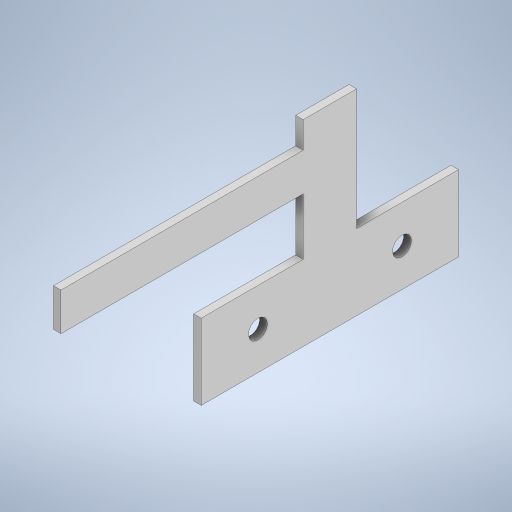
# Autodesk Inventor part: manual_locker_raw
Saved by Autodesk Inventor 2024 (Build 280153000, 153)
## iProperties
Created: 2025-12-30
Part Number: manual_locker_raw
Material: Generic
Document SubType Name: Modeling
Designer: schar
Density: 1 g/cm^3
Appearance: Default
Author: schar
Autodesk Inventor part; units mm, degrees
ref_plane "YZ Plane" through (0, 0, 0) normal (1, 0, 0) x (0, 1, 0)
ref_plane "XZ Plane" through (0, 0, 0) normal (0, 1, 0) x (-1, 0, 0)
ref_plane "XY Plane" through (0, 0, 0) normal (0, 0, 1) x (1, 0, 0)
sketch "Sketch1" plane through (0, 0, 0) normal (1, 0, 0) x (0, 1, 0)
  line L0 (10, 34.056) -> (-10, 34.056)
  line L1 (-10, 34.056) -> (-10, -34.056)
  line L2 (-10, -34.056) -> (10, -34.056)
  line L3 (10, -34.056) -> (10, 34.056)
  line L4 (10, 34.056) -> (-10, -34.056) construction
  line L5 (-10, 34.056) -> (10, -34.056) construction
  line L6 (10, 0) -> (10, -7.056)
  line L7 (10, -7.056) -> (42, -7.056)
  line L8 (42, -7.056) -> (42, 7.056)
  line L9 (42, 7.056) -> (10, 7.056)
  line L10 (10, 7.056) -> (10, -7.056)
  line L11 (0, 34.056) -> (0, 19.056)
  line L12 (0, -34.056) -> (0, -19.056)
  circle A0 centre (0, 19.056) radius 2.5
  circle A1 centre (0, -19.056) radius 2.5
  line L13 (10, 7.056) -> (10, 34.056)
  line L14 (10, 7.056) -> (10, 19.9232)
  line L15 (10, 19.9232) -> (25, 19.9232)
  line L16 (25, 19.9232) -> (25, 7.056)
  line L17 (25, 7.056) -> (10, 7.056)
  line L18 (25, 7.056) -> (25, 71.168)
  line L19 (25, 71.168) -> (35, 71.168)
  line L20 (35, 71.168) -> (35, 7.056)
  line L21 (35, 7.056) -> (25, 7.056)
  line L22 (35, 7.056) -> (35, 27.056)
  line L23 (35, 27.056) -> (25, 27.056)
  line L24 (35, 71.168) -> (35, 57.168)
  line L25 (35, 57.168) -> (25, 57.168)
  point P0 (0, 0)
  point P1 (0, 0)
  dimension "d0" = 20
  dimension "d1" = 68.112
  dimension "d2" = 7.056
  dimension "d3" = 32
  dimension "d4" = 14.112
  dimension "d5" = 15
  dimension "d6" = 15
  dimension "d7" = 5
  dimension "d8" = 5
  dimension "d9" = 15
  dimension "d10" = 64.112
  dimension "d11" = 10
  dimension "d12" = 20
  dimension "d13" = 14
  constraints: 52 end point, 8 parallel, 6 perpendicular, 5 midpoint, 5 point on line, 2 centre point, 2 coincident, 2 horizontal, 2 vertical
  measures "d0" distance of L2.end L2.start
  measures "d1" distance of L2.start L1.start
  measures "d2" distance of L6.start L6.end
  measures "d3" distance of L10.start L8.end
  measures "d4" distance of L8.end L7.end
  measures "d5" distance of L11.start L11.end
  measures "d6" distance of L12.start L12.end
  measures "d7" diameter of A0
  measures "d8" diameter of A1
  measures "d9" distance of L14.end L15.end
  measures "d10" distance of L19.end L20.end
  measures "d11" distance of L18.end L19.end
  measures "d12" distance of L20.end L22.end
  measures "d13" distance of L19.end L24.end
extrude "Extrusion1" add sketch "Sketch1" along normal blind 2 contours L3 L2 L1 L0 | L9 L8 L7 L3 | L18 L23 L20 L9 L16 | L18 L25 L20 L23 | L18 L19 L20 L25
body "Solid1"
